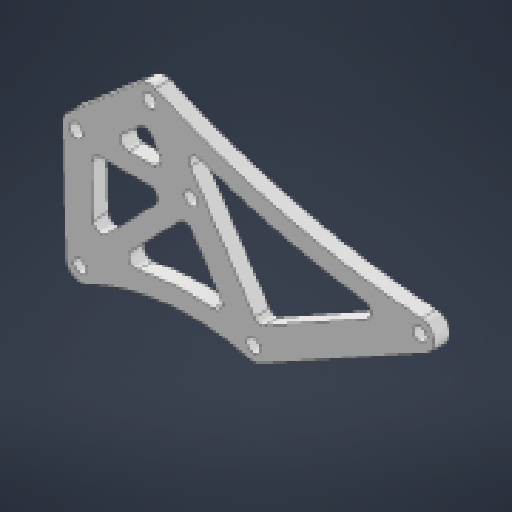
# Autodesk Inventor part: centralbrace
Saved by Autodesk Inventor 2025.2 (Build 292293000, 293)
## iProperties
Created: 2026-01-02
Part Number: centralbrace
Material: Acetal Resin, White
Document SubType Name: Modeling
Designer: cloudy
Density: 1.425 g/cm^3
Appearance: Smooth - Black
Author: cloudy
Autodesk Inventor part; units mm, degrees
ref_plane "YZ Plane" through (0, 0, 0) normal (1, 0, 0) x (0, 1, 0)
ref_plane "XZ Plane" through (0, 0, 0) normal (0, 1, 0) x (-1, 0, 0)
ref_plane "XY Plane" through (0, 0, 0) normal (0, 0, 1) x (1, 0, 0)
sketch "Sketch1" plane through (0, 0, 0) normal (0, 0, 1) x (1, 0, 0)
  circle A0 centre (10.765, 51.2851) radius 2.1844 projected
  circle A1 centre (31.5233, 19.3366) radius 2.1844 projected
  circle A2 centre (86.9588, 50.3069) radius 2.1844 projected
  circle A3 centre (-3.0738, 72.5841) radius 2.1844 projected
  circle A4 centre (-27.3318, 51.7742) radius 2.1844 projected
  circle A5 centre (-26.0367, 13.3556) radius 2.1844 projected
  arc A6 (30.2901, 14.7365) -> (33.8461, 15.1789) centre (31.5233, 19.3366) ccw
  arc A7 (89.2815, 46.1492) -> (87.0199, 55.069) centre (86.9588, 50.3069) ccw
  arc A8 (-1.1199, 76.9273) -> (-6.1747, 76.1988) centre (-3.0738, 72.5841) ccw
  arc A9 (-30.4327, 55.3889) -> (-32.0916, 51.6137) centre (-27.3318, 51.7742) ccw
  arc A10 (-30.7965, 13.1952) -> (-23.8841, 9.1074) centre (-26.0367, 13.3556) ccw
  line L0 (30.721, 29.3126) -> (6.3194, 66.8684)
  line L1 (-6.1747, 76.1988) -> (-30.4327, 55.3889)
  line L2 (-32.0916, 51.6137) -> (-30.7965, 13.1952)
  line L3 (33.8461, 15.1789) -> (89.2815, 46.1492)
  line L4 (-4.1028, 65.4266) -> (-16.8864, 54.4601)
  line L5 (9.1377, 45.0485) -> (-15.7743, 19.373)
  line L6 (3.2606, 48.1101) -> (-21.58, 22.5083)
  arc A11 (-1.1199, 76.9273) -> (87.2556, 55.0601) centre (103.0888, 308.5662) ccw
  arc A12 (30.2901, 14.7365) -> (-23.8841, 9.1074) centre (10.5583, -58.8644) ccw
  line L7 (3.0226, 54.4601) -> (-16.8864, 54.4601)
  line L8 (3.2606, 48.1101) -> (-22.4431, 48.1101)
  line L9 (75.984, 49.6309) -> (36.8851, 27.7874)
  arc A13 (23.7023, 22.6325) -> (-15.7743, 19.373) centre (10.5583, -58.8644) ccw
  line L10 (-21.58, 22.5083) -> (-22.4431, 48.1101)
  line L11 (23.7023, 22.6325) -> (9.1377, 45.0485)
  line L12 (3.0226, 54.4601) -> (-4.1028, 65.4266)
  line L13 (10.765, 51.2851) -> (-26.0367, 13.3556) construction
  line L14 (31.5233, 19.3366) -> (42.0802, 62.0019) construction
  line L15 (36.8851, 27.7874) -> (43.6417, 55.0939)
  line L16 (30.721, 29.3126) -> (37.4775, 56.6192)
  arc A14 (6.3194, 66.8684) -> (37.4775, 56.6192) centre (103.0888, 308.5662) ccw
  arc A15 (43.6417, 55.0939) -> (75.984, 49.6309) centre (103.0888, 308.5662) ccw
  point P0 (0, 0)
  dimension "d0" = 9.525
  dimension "d1" = 9.525
  dimension "d2" = 9.525
  dimension "d3" = 9.525
  dimension "d5" = 9.525
  dimension "d7" = 254
  dimension "d8" = 76.2
  dimension "d11" = 6.35
  dimension "d12" = 3.175
  dimension "d18" = 3.175
  dimension "d19" = 3.175
  dimension "d20" = 3.175
  dimension "d21" = 3.175
  dimension "d24" = 6.35
  constraints: 34 end point, 22 point on circle, 22 tangent, 10 centre point, 5 coincident, 5 parallel, 1 concentric, 1 horizontal, 1 other
  measures "d0" diameter of A6
  measures "d1" diameter of A7
  measures "d2" diameter of A8
  measures "d3" diameter of A9
  measures "d5" diameter of A10
  measures "d7" radius of A11
  measures "d8" radius of A12
  measures "d11" radial gap between concentric circles of A13 A12
  measures "d12" distance from line of L13.start L7
  measures "d18" distance from line of L13.start L8
  measures "d19" distance between parallel lines of L13 L5
  measures "d20" distance between parallel lines of L6 L13
  measures "d21" distance between parallel lines of L14 L15
  measures "d24" radial gap between concentric circles of A15 A11
extrude "Extrusion1" add sketch "Sketch1" along normal blind 6.35
fillet "Fillet1" radius 2.54 15 edges at (-15.7743, 19.373, 3.175) (9.1377, 45.0485, 3.175) (-4.1028, 65.4266, 3.175) (6.3194, 66.8684, 3.175) (3.2606, 48.1101, 3.175) (3.0226, 54.4601, 3.175) (-22.4431, 48.1101, 3.175) (-21.58, 22.5083, 3.175) (-16.8864, 54.4601, 3.175) (23.7023, 22.6325, 3.175) (75.984, 49.6309, 3.175) (43.6417, 55.0939, 3.175) (37.4775, 56.6192, 3.175) (30.721, 29.3126, 3.175) (36.8851, 27.7874, 3.175)
body "Solid1"
